M12_Camera_Mount_v2 (Autodesk Fusion 360 design; units mm, degrees)
Autodesk Fusion 360 part; units mm, degrees
sketch "Sketch2" plane through (0, 0, 0) normal (0, 0, 1) x (1, 0, 0)
  line L0 (8.5, -8.5) -> (-8.5, -8.5)
  line L1 (-8.5, -8.5) -> (-8.5, 8.5)
  line L2 (-8.5, 8.5) -> (8.5, 8.5)
  line L3 (8.5, 8.5) -> (8.5, -8.5)
  line L4 (8.5, -8.5) -> (-8.5, 8.5) construction
  line L5 (-8.5, -8.5) -> (8.5, 8.5) construction
  line L6 (8.5, 0) -> (9.8, 0) construction
  line L7 (8.5, -2.5) -> (9.8, -2.5)
  line L8 (8.5, 2.5) -> (9.8, 2.5)
  arc A0 (9.8, -2.5) -> (9.8, 2.5) centre (9.8, 0) ccw
  circle A1 centre (9.8, 0) radius 1
  line L9 (0, 0) -> (0, -8.5) construction
  circle A2 centre (-9.8, 0) radius 1
  line L10 (-8.5, -2.5) -> (-9.8, -2.5)
  line L11 (-8.5, 2.5) -> (-9.8, 2.5)
  arc A3 (-9.8, 2.5) -> (-9.8, -2.5) centre (-9.8, 0) ccw
  circle A4 centre (0, 0) radius 7.5
  circle A5 centre (0, 0) radius 6
  line L12 (1.25, -7.3951) -> (1.25, -8.5)
  line L13 (-1.25, -7.3951) -> (-1.25, -8.5)
  line L14 (7, -7) -> (-7, -7)
  line L15 (-7, -7) -> (-7, 7)
  line L16 (-7, 7) -> (7, 7)
  line L17 (7, 7) -> (7, -7)
  line L18 (7, -7) -> (-7, 7) construction
  line L19 (-7, -7) -> (7, 7) construction
  dimension "d1" = 17
  dimension "d2" = 17
  dimension "d4" = 1.3
  dimension "d5" = 2
  dimension "d6" = 15
  dimension "d7" = 12
  dimension "d8" = 1.25
  dimension "d9" = 14
  measures "d1" distance of L1.end L2.end
  measures "d2" distance of L0.end L1.end
  measures "d4" distance of L3 L6.end
  measures "d5" diameter of A1
  measures "d6" diameter of A4
  measures "d7" diameter of A5
  measures "d8" distance of L9 L12
  measures "d9" distance of L15.end L16.end
extrude "Extrude1" add sketch "Sketch2" along normal blind 8 contours L0 L1 L2 L3 A4 L12 L13 L14 L15 L16 L17 | L0 A4 L12 L13 | L3 L7 L8 A0 | A4 L14 | L1 L10 L11 A3 | A4 L17 | A4 L15 | A4 L16
extrude "Extrude2" add sketch "Sketch2" against normal blind 1.5 from surface at 8 contours A4 L14 L17 | A4 L14 L15 | A4 L16 L17 | A4 L15 L16
extrude "Extrude3" add sketch "Sketch2" along normal blind 6 and the other way blind 1.5 from surface at 8 contours L0 A4 L12 L13 | A4 L14 | A4 L14 L15 L16 L17 | A4 L17 | A4 L15 | A4 L16
extrude "Extrude4" cut 1 faces at (-0.1495, -6.6611, 6.5) along direction (0, 0, 1) blind 0.9
thread "Thread1" "ISO Metric profile 12.0 M12x0.5 6H" major diameter 12.0961 minor diameter 11.5287 pitch 0.5 angle 60 modelled right hand crest width 0.0625 on face at (5.9702, -0.5974, 9.6) crest through (5.7644, 0, 7.1188)
chamfer "Chamfer1" distance 0.5 angle 45 4 edges at (-10.7323, 0.3616, 8) (8.8677, 0.3616, 8) (8.8677, 0.3616, 0) (-10.7323, 0.3616, 0)
sketch "Sketch3" plane through (0, -8.5, 0) normal (0, -1, 0) x (1, 0, 0)
  line L0 (-1.25, 8) -> (-8.5, 8)
  line L1 (-8.5, 8) -> (-8.5, 0)
  line L2 (-8.5, 0) -> (8.5, 0)
  line L3 (8.5, 0) -> (8.5, 8)
  line L4 (8.5, 8) -> (1.25, 8)
  line L5 (1.25, 8) -> (1.25, 14)
  line L6 (1.25, 14) -> (-1.25, 14)
  line L7 (-1.25, 14) -> (-1.25, 8)
  line L8 (1.25, 11.9333) -> (-1.25, 11.9333) construction
  circle A0 centre (0, 11.9333) radius 0.5
  dimension "d23" = 1
  measures "d23" diameter of A0
extrude "Extrude5" cut sketch "Sketch3" against normal blind 4 contours A0
equation "d4 = 3.8 mm - 2.5 mm"
equation "d8 = ( 2.5 / 2 ) * 1 mm"
equation "d20 = -( 7.4 mm - 6.5 mm )"
named bodies: "M12 Camera Mount"
